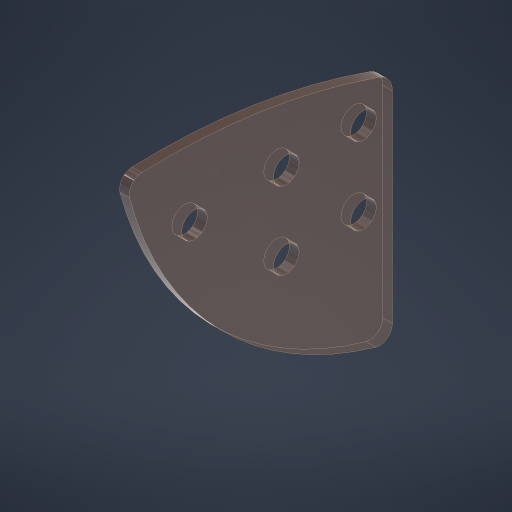
# Autodesk Inventor part: sled
Saved by Autodesk Inventor 2024 (Build 280153000, 153)
## iProperties
Created: 2023-08-09
Part Number: sled
Material: Polycarbonate, Smoke
Document SubType Name: Modeling
Designer: macbook
Density: 1.2 g/cm^3
Appearance: Polycarbonate - Smoked
Author: macbook
Autodesk Inventor part; units mm, degrees
ref_plane "YZ Plane" through (0, 0, 0) normal (1, 0, 0) x (0, 1, 0)
ref_plane "XZ Plane" through (0, 0, 0) normal (0, 1, 0) x (-1, 0, 0)
ref_plane "XY Plane" through (0, 0, 0) normal (0, 0, 1) x (1, 0, 0)
sketch "Sketch1" plane through (0, 0, 0) normal (1, 0, 0) x (0, 1, 0)
  line L0 (20.0034, -22.225) -> (-13.1281, -22.225)
  arc A0 (26.3176, 20.995) -> (-15.1614, -19.5199) centre (41.3356, -35.8708) ccw
  arc A1 (22.9977, -20.1059) -> (28.9733, 19.0246) centre (-77.1451, 15.2085) ccw
  arc A2 (28.9733, 19.0246) -> (26.3176, 20.995) centre (26.858, 18.9485) ccw
  arc A3 (-15.1614, -19.5199) -> (-13.1281, -22.225) centre (-13.1281, -20.1083) ccw
  arc A4 (20.0034, -22.225) -> (22.9977, -20.1059) centre (20.0034, -19.05) ccw
  point P0 (0, -22.225)
  point P1 (22.225, -22.225)
  point P2 (22.225, 18.2669)
  point P3 (-24.8206, -21.8938)
  point P4 (-15.875, -22.225)
  dimension "d1" = 22.225
  dimension "d55" = 38.1
  dimension "d57" = 2.1167
  dimension "d58" = 3.175
  constraints: 12 point on circle, 6 tangent, 5 centre point, 2 end point, 2 point on line, 1 equal radius, 1 horizontal
  measures "d1" distance of point (0, -22.225) point (22.225, -22.225)
  measures "d55" distance of point (22.225, -22.225) point (-15.875, -22.225)
  measures "d57" radius of A2
  measures "d58" radius of A4
extrude "Extrusion1" add sketch "Sketch1" along normal blind 1.5875
sketch "Sketch2" plane through (1.5875, 0, 0) normal (1, 0, 0) x (0, 0, -1)
  line L0 (22.225, 3.175) -> (22.225, 19.05) projected
  line L1 (0, 11.1125) -> (4.7625, 11.1125)
  line L2 (4.7625, 11.1125) -> (17.4625, 11.1125)
  line L3 (17.4625, 11.1125) -> (22.225, 11.1125)
  line L4 (4.7625, 11.1125) -> (4.7625, 17.4625)
  line L5 (17.4625, 17.4625) -> (17.4625, 4.7625)
  line L6 (4.7625, 4.7625) -> (4.7625, 11.1125)
  line L7 (4.7625, 17.4625) -> (-17.3369, 17.4625)
  line L8 (-19.3894, 19.515) -> (-0.8044, 0.9299) projected
  line L9 (-17.3369, 17.4625) -> (-13.9604, 20.8391)
  line L10 (-17.3369, 17.4625) -> (-12.5617, 17.4625) construction
  line L11 (-13.9604, 20.8391) -> (-6.7223, 13.601)
  line L12 (-13.9604, 20.8391) -> (-3.7242, 20.8391) construction
  point P0 (0, 0)
  point P1 (-10.3413, 17.22)
  dimension "d13" = 4.7625
  dimension "d14" = 12.7
  dimension "d15" = 6.35
  dimension "d16" = 12.7
  dimension "d49" = 4.7752
  dimension "d50" = 45
  dimension "d51" = 10.2362
  dimension "d52" = 45
  constraints: 22 end point, 4 coincident, 4 horizontal, 2 equal length, 2 midpoint, 2 vertical, 1 perpendicular, 1 point on line
  measures "d13" distance of L1.start L1.end
  measures "d14" distance of L1.end L2.end
  measures "d15" distance of L1.end L4.end
  measures "d16" distance of L5.start L5.end
  measures "d49" distance of L7.end L9.end
  measures "d50" angle of L10 L9
  measures "d51" distance of L9.end L11.end
  measures "d52" angle of L11 L12
hole "Hole1" at (1.5875, 17.4625, -4.7625) at (1.5875, 4.7625, -4.7625) at (1.5875, 17.22, 10.3413) at (1.5875, 17.4625, -17.4625) at (1.5875, 4.7625, -17.4625) direction (-1, 0, 0) diameter 4.2418 end through all
body "Solid1"
